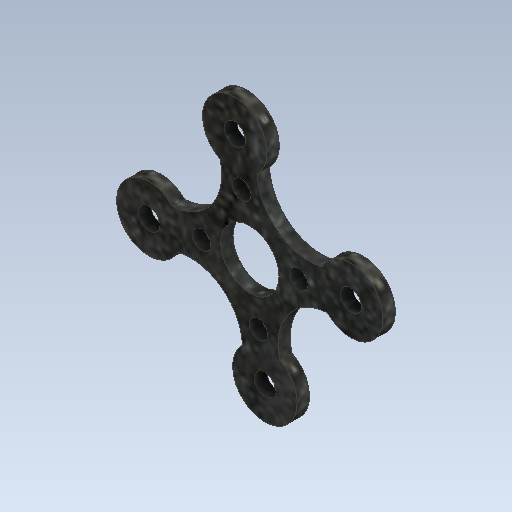
# Autodesk Inventor part: Part18
Saved by Autodesk Inventor 2021.1 (Build 251245010, 245A)
## iProperties
Created: 2023-10-20
Part Number: Part18
Material: Steel
Document SubType Name: Modeling
Designer: Lenovo
Density: 7.85 g/cm^3
Appearance: Plate
Mass: 8.07416 g
Surface Area: 15.8386 cm^2
Volume: 1.02856 cm^3
Author: Lenovo
Autodesk Inventor part; units mm, degrees
ref_plane "YZ Plane" through (0, 0, 0) normal (1, 0, 0) x (0, 1, 0)
ref_plane "XZ Plane" through (0, 0, 0) normal (0, 1, 0) x (-1, 0, 0)
ref_plane "XY Plane" through (0, 0, 0) normal (0, 0, 1) x (1, 0, 0)
sketch "Sketch1" plane through (0, 0, 0) normal (0, 0, 1) x (1, 0, 0)
  circle A0 centre (-12.4986, 205.4088) radius 1.5 projected
  circle A1 centre (-21.778, 213.3747) radius 1.5 projected
  circle A2 centre (-28.3229, 203.0439) radius 1.5 projected
  circle A3 centre (-19.0435, 195.0779) radius 1.5 projected
  arc A4 (-18.8621, 189.3065) -> (-17.5296, 189.5057) centre (-17.9571, 187.8087) ccw projected
  arc A5 (-5.4909, 205.775) -> (-5.6901, 207.1075) centre (-3.9931, 206.68) ccw projected
  arc A6 (-35.3306, 202.6777) -> (-35.1315, 201.3452) centre (-36.8284, 201.7727) ccw projected
  arc A7 (-21.9594, 219.1462) -> (-23.2919, 218.947) centre (-22.8644, 220.644) ccw projected
  arc A8 (-19.2274, 216.8536) -> (-8.6812, 209.0499) centre (-10.7552, 217.2751) ccw projected
  arc A9 (-33.0381, 205.4097) -> (-25.2343, 215.9559) centre (-33.4595, 213.8819) ccw projected
  arc A10 (-21.5941, 191.5991) -> (-32.1403, 199.4028) centre (-30.0663, 191.1776) ccw projected
  arc A11 (-7.7835, 203.043) -> (-15.5873, 192.4968) centre (-7.362, 194.5708) ccw projected
  circle A12 centre (-3.9931, 206.68) radius 5.2556
  circle A13 centre (-22.8644, 220.644) radius 5.2531
  circle A14 centre (-36.8284, 201.7727) radius 5.2531
  circle A15 centre (-17.9571, 187.8087) radius 5.2531
  circle A16 centre (-3.9931, 206.68) radius 1.75
  circle A17 centre (-22.8644, 220.644) radius 1.75
  circle A18 centre (-36.8284, 201.7727) radius 1.75
  circle A19 centre (-17.9571, 187.8087) radius 1.75
  circle A20 centre (-20.4108, 204.2263) radius 4.75 projected
  point P0 (0, 0)
  point P1 (-18.8621, 189.3065)
  point P2 (-17.5296, 189.5057)
  point P3 (-21.9594, 219.1462)
  point P4 (-23.2919, 218.947)
  point P5 (-5.4909, 205.775)
  point P6 (-5.6901, 207.1075)
  point P7 (-32.1403, 199.4028)
  point P8 (-21.5941, 191.5991)
  point P9 (-7.7868, 203.0428)
  point P10 (-8.6845, 209.0491)
  point P11 (-25.2343, 215.9559)
  constraints: 9 coincident, 6 centre point, 3 concentric, 6 other
extrude "Extrusion1" add sketch "Sketch1" along normal blind 2
body "Solid1"
